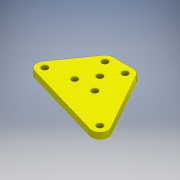
# Autodesk Inventor part: LegBase_front
Saved by Autodesk Inventor 2016 (Build 200138000, 138)
## iProperties
Created: 2015-12-07
Part Number: LegBase_front
Material: Generic
Document SubType Name: Modeling
Designer: lk8187
Density: 1 g/cm^3
Appearance: Smooth - Yellow
Author: lk8187
Autodesk Inventor part; units mm, degrees
ref_plane "YZ Plane" through (0, 0, 0) normal (1, 0, 0) x (0, 1, 0)
ref_plane "XZ Plane" through (0, 0, 0) normal (0, 1, 0) x (-1, 0, 0)
ref_plane "XY Plane" through (0, 0, 0) normal (0, 0, 1) x (1, 0, 0)
sketch "Sketch1" plane through (0, 0, 0) normal (0, 0, 1) x (1, 0, 0)
  line L0 (5, -7.5) -> (-5, -7.5) construction
  line L1 (-5, -7.5) -> (-5, 7.5) construction
  line L2 (-5, 7.5) -> (5, 7.5) construction
  line L3 (5, 7.5) -> (5, -7.5) construction
  line L4 (5, -7.5) -> (-5, 7.5) construction
  line L5 (-5, -7.5) -> (5, 7.5) construction
  line L6 (0, 0) -> (21.2132, -21.2132) construction
  line L7 (0, 0) -> (-17.3205, -10) construction
  line L8 (-20.5912, -7.6973) -> (-8.2707, 9.8027)
  arc A0 (-5, 11.5) -> (-8.2707, 9.8027) centre (-5, 7.5) ccw
  line L9 (-5, 11.5) -> (5, 11.5)
  arc A1 (8.4831, 9.4668) -> (5, 11.5) centre (5, 7.5) ccw
  line L10 (8.4831, 9.4668) -> (24.6963, -19.2464)
  arc A2 (20.0956, -25.0539) -> (24.6963, -19.2464) centre (21.2132, -21.2132) ccw
  line L11 (20.0956, -25.0539) -> (-18.4381, -13.8407)
  arc A3 (-20.5912, -7.6973) -> (-18.4381, -13.8407) centre (-17.3205, -10) ccw
  dimension "d0" = 10
  dimension "d1" = 15
  dimension "d2" = 30
  dimension "d4" = 45
  dimension "d5" = 30
  dimension "d6" = 20
  dimension "d7" = 4
  constraints: 24 end point, 11 coincident, 8 point on circle, 8 tangent, 4 centre point, 3 equal radius, 2 midpoint, 2 parallel, 1 horizontal, 1 perpendicular
  measures "d0" distance of L1.end L2.end
  measures "d1" distance of L0.end L1.end
  measures "d2" distance of L6.start L6.end
  measures "d4" angle of L0 L6
  measures "d5" angle of L0 L7
  measures "d6" distance of L6.start L7.end
  measures "d7" radius of A0
extrude "Extrusion1" add sketch "Sketch1" against normal blind 3
hole "Hole1" at (-5, 7.5, 0) at (5, 7.5, 0) at (5, -7.5, 0) at (-5, -7.5, 0) direction (0, 0, -1) diameter 3 depth 8 tip angle 118
hole "Hole2" at (-17.3205, -10, 0) at (21.2132, -21.2132, 0) direction (0, 0, -1) diameter 3 depth 8 tip angle 118
hole "Hole3" at (0, 0, 0) direction (0, 0, -1) diameter 3 depth 8 tip angle 118
body "Solid1"
